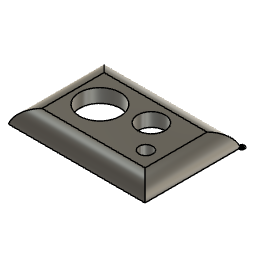
keychain_lab1homework v1 (Autodesk Fusion 360 design; units mm, degrees)
Autodesk Fusion 360 part; units mm, degrees
sketch "Sketch1" plane through (0, 0, 0) normal (0, 0, 1) x (1, 0, 0)
  line L0 (-50, 25) -> (50, 25)
  line L1 (50, 25) -> (50, -45)
  line L2 (50, -45) -> (-50, -45)
  line L3 (-50, -45) -> (-50, 25)
  dimension "d1" = 100
  dimension "d2" = 70
  constraint vertical L1
  constraint horizontal L2
  constraint vertical L3
  measures "d1" distance of L0.start L0.end
  measures "d2" distance of L0.start L2.end
extrude "Extrude1" add sketch "Sketch1" along normal blind 10
fillet "Fillet1" radius 12.5 4 edges at (-50, -10, 10) (50, -10, 10) (0, -45, 10) (0, 25, 10)
hole "Hole1" at (26.7973, -21.1213, 10) direction (0, 0, -1) diameter 10 depth 30 tip angle 118
hole "Hole2" at (11.4224, -1.7527, 10) direction (0, 0, -1) diameter 20 depth 30 tip angle 118
hole "Hole3" at (-0.688, -19.8131, 10) direction (0, 0, -1) diameter 10 depth 30 tip angle 118
delete_face "DeleteFace1" 1 faces at (-0.4388, -24.8069, 6.6667)
sketch "Sketch2" plane through (0, 0, 0) normal (0, 0, 1) x (1, 0, 0)
  circle A0 centre (50.3697, 25.69) radius 2
  dimension "d15" = 4
  measures "d15" diameter of A0
extrude "Extrude2" add sketch "Sketch2" along normal blind 0.5
hole "Hole4" at (50.4116, 25.8445, 0.5) direction (0, 0, -1) diameter 2 depth 30 tip angle 118
hole "Hole5" at (-19.1275, -8.9179, 10) direction (0, 0, -1) diameter 30 depth 30 tip angle 118
